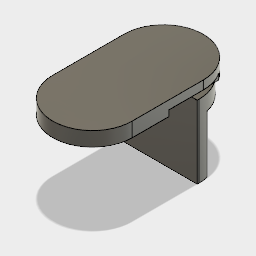
servo_bracket_elbow_2 (Autodesk Fusion 360 design; units mm, degrees)
Autodesk Fusion 360 part; units mm, degrees
sketch "スケッチ1" plane through (0, 0, 0) normal (0, 1, 0) x (1, 0, 0)
  line L0 (0, 0) -> (14.3, 0)
  line L1 (14.3, 0) -> (14.3, -12.8)
  line L2 (14.3, -12.8) -> (0, -12.8)
  line L3 (0, -12.8) -> (0, 0)
  circle A0 centre (7.15, 0) radius 7.15
  circle A1 centre (7.15, -12.8) radius 7.15
  dimension "d1" = 14.3
  dimension "d2" = 12.8
  constraint horizontal L0
  constraint vertical L1
  constraint horizontal L2
  constraint vertical L3
  constraint coincident A0
  constraint tangent L1 A0
  constraint coincident A1
  constraint tangent L1 A1
extrude "押し出し1" add sketch "スケッチ1" along normal blind 2.6
sketch "スケッチ2" plane through (0, 0, 0) normal (0, 1, 0) x (1, 0, 0)
  line L0 (7.15, 0) -> (7.15, -0.786)
  line L1 (7.15, 0) -> (7.936, 0) construction
  circle A0 centre (7.15, -0.786) radius 7.15
  arc A1 (14.3, 0) -> (0, 0) centre (7.15, 0) ccw
  line L2 (7.15, 7.15) -> (7.15, 0.9)
  line L3 (7.15, 7.15) -> (13.4, 7.15) construction
  line L4 (7.15, 0.9) -> (0.2016, 0.9)
  line L5 (7.15, 0.9) -> (14.0984, 0.9)
  line L6 (7.15, 0.9) -> (7.15, -1.1)
  line L7 (7.15, 0.9) -> (9.15, 0.9) construction
  line L8 (14.3, -12.8) -> (14.3, 0)
  line L9 (7.15, -1.1) -> (14.2931, -1.1)
  line L10 (0, 0) -> (0, -12.8)
  line L11 (7.15, -1.1) -> (14.2931, -1.1) construction
  line L12 (14.3, 0) -> (14.3, -12.8)
  line L13 (14.2931, -1.1) -> (14.3, -1.1)
  line L14 (0.0069, -1.1) -> (0, -1.1)
  line L15 (0.0069, -1.1) -> (0.0138, -1.1) construction
  line L16 (0, -12.8) -> (0, 0)
  line L17 (7.15, -1.1) -> (0, -1.1)
  line L18 (7.15, -1.1) -> (14.3, -1.1)
  line L19 (14.3, -1.1) -> (14.3, -0.786)
  line L20 (0, -1.1) -> (0, -0.786)
  dimension "d5" = 90
  dimension "d6" = 0.786
  dimension "d7" = 14.3
  dimension "d8" = 90
  dimension "d9" = 6.25
  dimension "d10" = 90
  dimension "d11" = 2
  dimension "d20" = 180
  constraint horizontal L1
  constraint midpoint A1
  constraint horizontal L3
  constraint coincident A0
  constraint perpendicular L2 L4
  constraint perpendicular L2 L5
  constraint horizontal L7
  constraint perpendicular L8 L9
  constraint horizontal L11
  constraint coincident L8
  constraint coincident L10
  constraint horizontal L15
  constraint perpendicular L16 L17
  constraint perpendicular L12 L18
  constraint tangent A0 L19
  constraint tangent A0 L20
  measures "d5" angle of L0 L1
  measures "d7" diameter of A0
  measures "d8" angle of L2 L3
  measures "d10" angle of L6 L7
  measures "d20" angle of L14 L15
extrude "押し出し2" add sketch "スケッチ2" against normal blind 3.8 contours A0 L2 L4 | A0 L2 L5
extrude "押し出し5" add sketch "スケッチ2" against normal blind 14.15 contours L0 A0 L5 L6 L9 L18 | L0 A0 L4 L6 L17 | A0 L8 L12 L13 L18 L19 | A0 L10 L14 L16 L17 L20
sketch "スケッチ3" plane through (0, 0, 0) normal (0, 1, 0) x (1, 0, 0)
  circle A0 centre (7.15, -12.8) radius 2
  dimension "d17" = 4
  measures "d17" diameter of A0
extrude "押し出し4" cut sketch "スケッチ3" along normal blind 2
ref_plane "作業平面2" through (7.15, -7.075, 1.1) normal (0, 0, 1) x (-1, 0, 0)
sketch "スケッチ4" plane through (7.15, -7.075, 1.1) normal (0, 0, 1) x (1, 0, 0)
  line L0 (-7.15, 7.075) -> (-5.95, 7.075)
  line L1 (-5.95, 7.075) -> (-5.95, 6.075)
  line L2 (-5.95, 6.075) -> (-7.15, 6.075)
  line L3 (-7.15, 6.075) -> (-7.15, 7.075)
  line L4 (7.15, 7.075) -> (5.95, 7.075)
  line L5 (5.95, 7.075) -> (5.95, 6.075)
  line L6 (5.95, 6.075) -> (7.15, 6.075)
  line L7 (7.15, 6.075) -> (7.15, 7.075)
  dimension "d24" = 1
  dimension "d25" = 1.2
  dimension "d26" = 1.2
  dimension "d27" = 1
  constraint horizontal L0
  constraint vertical L1
  constraint horizontal L2
  constraint vertical L3
  constraint horizontal L4
  constraint vertical L5
  constraint horizontal L6
  constraint vertical L7
extrude "押し出し6" cut sketch "スケッチ4" against normal blind 11.5
sketch "スケッチ5" plane through (0, 0, 0) normal (0, -1, 0) x (1, 0, 0)
  line L0 (1.2, 1.1) -> (13.1, 1.1)
  line L1 (13.1, 1.1) -> (13.1, -3.1788)
  arc A0 (1.2, -3.1788) -> (13.1, -3.1788) centre (7.15, 0.786) ccw
  line L2 (1.2, -3.1788) -> (1.2, 1.1)
  circle A1 centre (7.15, 12.8) radius 2
  line L3 (0, 12.8) -> (0, 0)
  arc A2 (0, 0) -> (14.3, 0) centre (7.15, 0) ccw
  line L4 (14.3, 0) -> (14.3, 12.8)
  arc A3 (14.3, 12.8) -> (0, 12.8) centre (7.15, 12.8) ccw
  line L5 (13.1, 1.1) -> (13.1, 6.2)
  line L6 (13.1, 1.1) -> (13.1, -3.1788)
  line L7 (14.3, 1.1) -> (14.3, 6.2)
  line L8 (13.1, 6.2) -> (14.3, 6.2)
  line L9 (1.2, 1.1) -> (1.2, 6.2)
  line L10 (0, 1.1) -> (0, 6.2)
  line L11 (1.2, 6.2) -> (0, 6.2)
  circle A4 centre (7.15, 0) radius 7.15
  line L12 (1.2, 1.1) -> (1.2131, -3.9844)
  line L13 (13.1, 1.1) -> (13.092, -3.9768)
  dimension "d30" = 5.1
  dimension "d31" = 5.1
  dimension "d32" = 5.1
  dimension "d33" = 5.1
  constraint perpendicular L7 L8
  constraint perpendicular L10 L11
  constraint concentric A2 A4
  constraint coincident A4
  constraint coincident A2
extrude "押し出し7" cut sketch "スケッチ5" against normal blind 1.05 contours A0 L2 A2 L9 A4 L12 | L1 A0 A2 L5 L6 A4 L13 | L3 L9 L10 L11 A4 | L4 L5 L7 L8 A4
extrude "押し出し8" add 2 faces at (0.4257, -1, 0.5417) (13.8743, -1, 0.5417) along direction (0, 1, 0) blind 1
extrude "押し出し9" [suppressed]
extrude "押し出し10" cut 1 faces at (4.9905, -3.8, -1.8871) along direction (0, 1, 0) blind 1
extrude "押し出し11" cut 1 faces at (9.4661, -14.15, 0.224) along direction (0, 1, 0) blind 1.05
equation "d42 = -14.15 mm + 13.3 mm - 0.2 mm"
